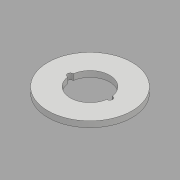
# Autodesk Inventor part: 銅墊塊-50T
Saved by Autodesk Inventor 2018 (Build 220112000, 112)
## iProperties
Created: 2023-03-17
Part Number: 銅墊塊-50T
Material: 一般
Document SubType Name: Modeling
Designer: chihhao
Density: 1 g/cm^3
Appearance: 預設
Author: chihhao
Autodesk Inventor part; units mm, degrees
ref_plane "YZ Plane" through (0, 0, 0) normal (1, 0, 0) x (0, 1, 0)
ref_plane "XZ Plane" through (0, 0, 0) normal (0, 1, 0) x (-1, 0, 0)
ref_plane "XY Plane" through (0, 0, 0) normal (0, 0, 1) x (1, 0, 0)
sketch "草圖1" plane through (0, 0, 0) normal (0, 0, 1) x (1, 0, 0)
  circle A0 centre (0, 0) radius 32
  dimension "d0" = 64
  constraints: 1 centre point, 1 coincident
  measures "d0" diameter of A0
extrude "擠出1" add sketch "草圖1" along normal blind 4.5
sketch "草圖2" plane through (0, 0, 4.5) normal (0, 0, 1) x (1, 0, 0)
  point P0 (0, 0)
  point P1 (0, 0)
  constraints: 1 coincident
hole "孔1" at (0, 0, 4.5) direction (0, 0, -1) diameter 30 end through all
sketch "草圖3" plane through (0, 0, 4.5) normal (0, 0, 1) x (1, 0, 0)
  circle A0 centre (15, 0) radius 2.15
  point P0 (0, 0)
  dimension "d10" = 0
  dimension "d11" = 4.3
  dimension "d12" = 15
  constraints: 1 centre point
  measures "d10" vertical distance of point (0, 0) A0.centre
  measures "d11" diameter of A0
  measures "d12" distance of point (0, 0) A0.centre
extrude "擠出2" cut sketch "草圖3" against normal blind 20
pattern_circular "環形陣列1" count 2 over 360 about axis through (0, 0, -86.1215) along (0, 0, 1) of "擠出2"
